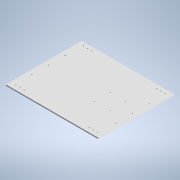
# Autodesk Inventor part: 000.001 - Bottom
Saved by Autodesk Inventor 2022 (Build 260153000, 153)
## iProperties
Created: 2021-06-26
Part Number: 000.001 - Bottom
Material: Типовые
Document SubType Name: Modeling
Designer: Петров Иван
Mass: 118.121 g
Surface Area: 818.262 cm^2
Volume: 118.121 cm^3
Density: 1 g/cm^3
Appearance: По умолчанию
Author: Петров Иван
Autodesk Inventor part; units mm, degrees
ref_plane "YZ Plane" through (0, 0, 0) normal (1, 0, 0) x (0, 1, 0)
ref_plane "XZ Plane" through (0, 0, 0) normal (0, 1, 0) x (-1, 0, 0)
ref_plane "XY Plane" through (0, 0, 0) normal (0, 0, 1) x (1, 0, 0)
sketch "Эскиз1" plane through (0, 0, 0) normal (0, 1, 0) x (-1, 0, 0)
  line L0 (-110, 90) -> (110, 90)
  line L1 (110, 90) -> (110, -90)
  line L2 (110, -90) -> (-110, -90)
  line L3 (-110, -90) -> (-110, 90)
  line L4 (-110, 90) -> (110, -90) construction
  line L5 (110, 90) -> (-110, -90) construction
  point P0 (0, 0)
  dimension "d0" = 220
  dimension "d1" = 180
  constraints: 12 end point, 2 midpoint, 2 parallel, 1 horizontal, 1 perpendicular
  measures "d0" distance of L1.end L2.end
  measures "d1" distance of L0.end L1.end
extrude "Выдавливание1" add sketch "Эскиз1" along normal blind 3
sketch "Эскиз4" plane through (0, 0, 0) normal (0, -1, 0) x (1, 0, 0)
  circle A0 centre (99.9996, -40) radius 2 projected
  circle A1 centre (99.9996, 0) radius 2 projected
  circle A2 centre (99.9996, 40) radius 2 projected
  circle A3 centre (-99.9997, 0) radius 2 projected
  circle A4 centre (-99.9997, -40) radius 2 projected
  circle A5 centre (-99.9997, 40) radius 2 projected
  point P0 (0, 0)
extrude "Выдавливание4" cut sketch "Эскиз4" against normal blind 3
sketch "Эскиз5" plane through (0, 0, 0) normal (0, -1, 0) x (1, 0, 0)
  circle A0 centre (-97.5, 80.5) radius 2 projected
  circle A1 centre (-87.5, 80.5) radius 2 projected
  circle A2 centre (-77.5, 80.5) radius 2 projected
  circle A3 centre (-97.5, -80.5) radius 2 projected
  circle A4 centre (-87.5, -80.5) radius 2 projected
  circle A5 centre (-77.5, -80.5) radius 2 projected
  circle A6 centre (77.5, -80.5) radius 2 projected
  circle A7 centre (87.5, -80.5) radius 2 projected
  circle A8 centre (97.5, -80.5) radius 2 projected
  circle A9 centre (87.5, 80.5) radius 2 projected
  circle A10 centre (97.5, 80.5) radius 2 projected
  circle A11 centre (77.5, 80.5) radius 2 projected
  point P0 (0, 0)
extrude "Выдавливание5" cut sketch "Эскиз5" against normal blind 10
sketch "Эскиз6" plane through (0, 3, 0) normal (0, 1, 0) x (1, 0, 0)
  circle A0 centre (66.6857, -20.1363) radius 1.75 projected
  circle A1 centre (29.9439, -20.1363) radius 1.75 projected
  circle A2 centre (29.9439, 17.2432) radius 1.75 projected
  circle A3 centre (66.6857, 17.2432) radius 1.75 projected
  point P0 (0, 0)
extrude "Выдавливание6" cut sketch "Эскиз6" against normal blind 10
